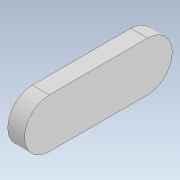
# Autodesk Inventor part: shank_board
Saved by Autodesk Inventor 2020 (Build 240168000, 168)
## iProperties
Created: 2021-01-12
Part Number: shank_board
Material: Generic
Document SubType Name: Modeling
Designer: DELL
Density: 1 g/cm^3
Appearance: Default
Author: DELL
Autodesk Inventor part; units mm, degrees
ref_plane "YZ Plane" through (0, 0, 0) normal (1, 0, 0) x (0, 1, 0)
ref_plane "XZ Plane" through (0, 0, 0) normal (0, 1, 0) x (-1, 0, 0)
ref_plane "XY Plane" through (0, 0, 0) normal (0, 0, 1) x (1, 0, 0)
sketch "Sketch1" plane through (0, 0, 0) normal (1, 0, 0) x (0, 1, 0)
  circle A0 centre (0, 0) radius 17.5
  circle A1 centre (0, -70) radius 17.5
  line L0 (-17.5, 0) -> (-17.5, -70)
  line L1 (17.5, 0) -> (17.5, -70)
  dimension "d0" = 35
  dimension "d1" = 70
  constraints: 4 end point, 4 point on circle, 4 tangent, 2 centre point, 1 coincident, 1 equal radius, 1 vertical alignment
  measures "d0" diameter of A0
  measures "d1" distance of L1.start L1.end
extrude "Extrusion1" add sketch "Sketch1" along normal blind 12
body "Solid1"
